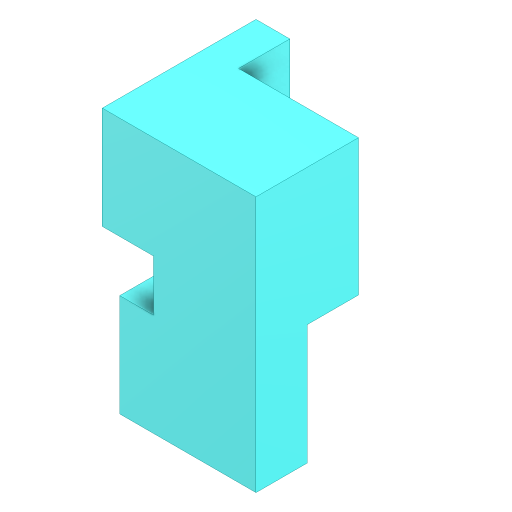
# Autodesk Inventor part: support_ladder
Saved by Autodesk Inventor 2024 (Build 280153000, 153)
## iProperties
Created: 2024-06-06
Part Number: support_ladder
Material: 一般
Document SubType Name: Modeling
Designer: admin
Density: 1 g/cm^3
Appearance: 平滑 - 灰白色
Author: admin
Autodesk Inventor part; units mm, degrees
ref_plane "YZ Plane" through (0, 0, 0) normal (1, 0, 0) x (0, 1, 0)
ref_plane "XZ Plane" through (0, 0, 0) normal (0, 1, 0) x (-1, 0, 0)
ref_plane "XY Plane" through (0, 0, 0) normal (0, 0, 1) x (1, 0, 0)
sketch "草圖2" plane through (0, 0, 0) normal (0, 0, 1) x (1, 0, 0)
  line L0 (5, -5) -> (-5, -5)
  line L1 (-5, -5) -> (-5, 5)
  line L2 (-5, 5) -> (5, 5)
  line L3 (5, 5) -> (5, -5)
  line L4 (5, -5) -> (-5, 5) construction
  line L5 (-5, -5) -> (5, 5) construction
  line L6 (25, -25) -> (-25, -25)
  line L7 (-25, -25) -> (-25, 25)
  line L8 (-25, 25) -> (25, 25)
  line L9 (25, 25) -> (25, -25)
  line L10 (25, -25) -> (-25, 25) construction
  line L11 (-25, -25) -> (25, 25) construction
  line L12 (-25, -25) -> (-1.6, -25)
  line L13 (-1.6, -25) -> (-1.6, -5)
  line L14 (-1.6, -5) -> (-25, -5)
  line L15 (-25, -5) -> (-25, -25)
  line L16 (25, -25) -> (-4.3496, -25)
  line L17 (-4.3496, -5) -> (25, -5)
  line L18 (25, -5) -> (25, -25)
  line L19 (25, -25) -> (5, -25)
  line L20 (5, -25) -> (5, -1.6)
  line L21 (5, -1.6) -> (25, -1.6)
  line L22 (25, -1.6) -> (25, -25)
  line L23 (25, 25) -> (5, 25)
  line L24 (5, 25) -> (5, 5.2641)
  line L25 (25, 5.2641) -> (25, 25)
  line L26 (25, 25) -> (1.6, 25)
  line L27 (1.6, 25) -> (1.6, 5)
  line L28 (1.6, 5) -> (25, 5)
  line L29 (25, 5) -> (25, 25)
  line L30 (-25, 25) -> (-1.1496, 25)
  line L31 (-1.1496, 5) -> (-25, 5)
  line L32 (-25, 5) -> (-25, 25)
  line L33 (-5, -5) -> (-25, -5)
  line L34 (-25, -5) -> (-25, -25)
  line L35 (-25, -25) -> (-5, -25)
  line L36 (-5, -25) -> (-5, -5)
  line L37 (-1.6, -25) -> (-13.2, -25)
  line L38 (-13.2, -25) -> (-13.2, -5)
  line L39 (-13.2, -5) -> (-1.6, -5)
  line L40 (-1.6, -5) -> (-1.6, -25)
  line L41 (5, -1.6) -> (25, -1.6)
  line L42 (25, -1.6) -> (25, -13.2)
  line L43 (25, -13.2) -> (5, -13.2)
  line L44 (5, -13.2) -> (5, -1.6)
  line L45 (1.6, 5) -> (13.2, 5)
  line L46 (13.2, 5) -> (13.2, 25)
  line L47 (13.2, 25) -> (1.6, 25)
  line L48 (1.6, 25) -> (1.6, 5)
  line L49 (1.6, 5) -> (-5, 5)
  line L50 (-5, 5) -> (-5, 25)
  line L51 (-5, 25) -> (1.6, 25)
  line L52 (1.6, 25) -> (1.6, 5)
  point P0 (0, 0)
  point P1 (0, 0)
  point P2 (0, 0)
  point P3 (-4.3496, -18.1359)
  point P4 (-7.7496, 1.8641)
  point P5 (-27.7496, 1.8641)
  point P6 (22.2504, 5.2641)
  point P7 (2.2504, 1.8641)
  point P8 (2.2504, -18.1359)
  point P9 (-7.7496, 1.8641)
  point P10 (2.2504, 1.8641)
  point P11 (-1.1496, 31.8641)
  point P12 (-27.7496, 11.8641)
  point P13 (-7.7496, 11.8641)
  point P14 (-1.1496, 11.8641)
  point P15 (-7.7496, 11.8641)
  point P16 (2.2504, 1.8641)
  point P17 (22.2504, 1.8641)
  point P18 (-7.7496, -18.1359)
  point P19 (2.2504, 11.8641)
  point P20 (2.2504, 31.8641)
  point P21 (-1.1496, 31.8641)
  point P22 (-7.7496, -18.1359)
  point P23 (-15.9496, 1.8641)
  point P24 (-15.9496, -18.1359)
  point P25 (-7.7496, 1.8641)
  point P26 (2.2504, -6.3359)
  point P27 (22.2504, -6.3359)
  point P28 (-7.7496, 31.8641)
  point P29 (-7.7496, 11.8641)
  point P30 (2.2504, 11.8641)
  point P31 (10.4504, 11.8641)
  point P32 (10.4504, 31.8641)
  point P33 (-1.6, -25)
  point P34 (-5, 5)
  dimension "d13" = 10
  dimension "d14" = 20
  dimension "d15" = 1.6
  dimension "d16" = 1.6
  dimension "d17" = 1.6
  dimension "d18" = 0
  dimension "d19" = 11.6
  dimension "d20" = 11.6
  dimension "d21" = 11.6
  dimension "d22" = 10
  constraints: 106 end point, 23 parallel, 13 horizontal, 13 perpendicular, 11 point on line, 4 midpoint, 2 coincident
  measures "d13" distance of L1.end L2.end
  measures "d14" distance between parallel lines of L8 L2
  measures "d15" distance from line of point (0, 0) L13
  measures "d16" distance from line of point (0, 0) L21
  measures "d17" distance from line of point (0, 0) L27
  measures "d18" distance between parallel lines of L7 L32
  measures "d19" distance between parallel lines of L38 L13
  measures "d20" distance between parallel lines of L41 L43
  measures "d21" distance between parallel lines of L27 L46
  measures "d22" distance between parallel lines of L50 L24
extrude "擠出1" add sketch "草圖2" against normal blind 10 contours L20 L6 L13 L0 | L3 L21 L9 L17 | L17 L9 L43 L20 | L43 L9 L6 L20
extrude "擠出2" add sketch "草圖2" against normal blind 20 contours L3 L28 L9 L21 | L2 L27 L8 L46 L28 | L46 L8 L9 L28
extrude "擠出3" add sketch "草圖2" against normal blind 30 contours L2 L50 L8 L27
equation "\"d14\" = d23"
equation "\"d15\" = d24"
equation "\"d16\" = d24"
equation "\"d17\" = d24"
equation "\"d19\" = d25"
equation "\"d20\" = d25"
equation "\"d21\" = d25"
equation "\"d11\" = 1.6"
equation "\"d12\" = 11.6"
equation "\"d23\" = 20"
equation "\"d24\" = 1.6"
equation "\"d25\" = 11.6"
